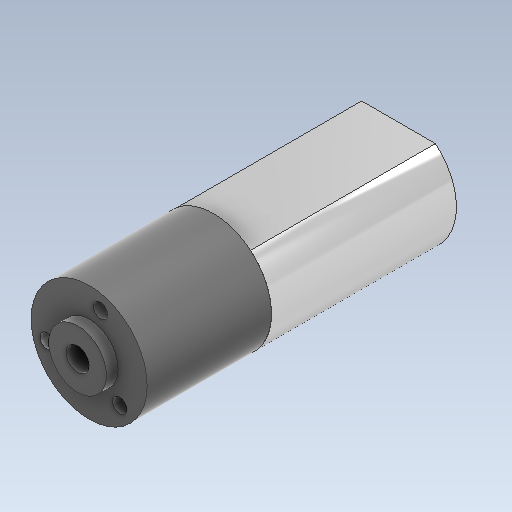
# Autodesk Inventor part: motor_body
Saved by Autodesk Inventor 2020 (Build 240168000, 168)
## iProperties
Created: 2023-12-19
Part Number: motor_body
Material: Типовые
Document SubType Name: Modeling
Designer: denis
Density: 1 g/cm^3
Appearance: По умолчанию
Author: denis
Autodesk Inventor part; units mm, degrees
ref_plane "YZ Plane" through (0, 0, 0) normal (1, 0, 0) x (0, 1, 0)
ref_plane "XZ Plane" through (0, 0, 0) normal (0, 1, 0) x (-1, 0, 0)
ref_plane "XY Plane" through (0, 0, 0) normal (0, 0, 1) x (1, 0, 0)
sketch "Эскиз1" plane through (0, 0, 0) normal (0, 0, 1) x (1, 0, 0)
  circle A0 centre (0, 0) radius 10.025
  dimension "d0" = 20.05
  constraints: 1 centre point, 1 coincident
  measures "d0" diameter of A0
extrude "Выдавливание1" add sketch "Эскиз1" along normal blind 21.5
sketch "Эскиз2" plane through (0, 0, 21.5) normal (0, 0, 1) x (1, 0, 0)
  circle A0 centre (0, 0) radius 5
  dimension "d3" = 10
  constraints: 1 centre point, 1 coincident
  measures "d3" diameter of A0
extrude "Выдавливание2" add sketch "Эскиз2" along normal blind 2
sketch "Эскиз3" plane through (0, 0, 0) normal (0, 0, -1) x (-1, 0, 0)
  circle A0 centre (0, 0) radius 10
  line L0 (6.3804, -7.7) -> (-6.4196, -7.7)
  circle A1 centre (0, 0) radius 10.025 construction
  line L1 (-10.025, 0) -> (10.025, 0) construction
  circle A2 centre (0, 0) radius 10.025 construction
  line L2 (6.3804, 7.7) -> (-6.4196, 7.7)
  point P0 (-6.3804, 7.7)
  point P1 (-6.3804, -7.7)
  dimension "d6" = 20
  dimension "d10" = 15.4
  constraints: 6 end point, 5 point on circle, 2 horizontal, 2 symmetric about line, 1 centre point, 1 coincident
  measures "d6" diameter of A0
  measures "d10" distance between parallel lines of L0 L2
extrude "Выдавливание3" add sketch "Эскиз3" along normal blind 32 contours A0 L0 L2
sketch "Эскиз4" plane through (0, 0, 21.5) normal (0, 0, 1) x (1, 0, 0)
  circle A0 centre (0, 0) radius 7.5 construction
  circle A1 centre (1.9411, 7.2444) radius 1.25
  circle A2 centre (0, 0) radius 10.025 construction
  line L0 (0, 10.025) -> (0, -10.025) construction
  line L1 (1.9411, 7.2444) -> (0, 0) construction
  circle A3 centre (-7.2444, -1.9411) radius 1.25
  circle A4 centre (5.3033, -5.3033) radius 1.25
  dimension "d11" = 15
  dimension "d12" = 2.5
  dimension "d13" = 15
  dimension "d16" = 360
  constraints: 4 end point, 3 centre point, 2 point on circle, 2 vertical, 1 coincident, 10 other
  measures "d12" diameter of A1
  measures "d13" angle of L0 L1
extrude "Выдавливание4" cut sketch "Эскиз4" against normal blind 5
sketch "Эскиз5" plane through (0, 0, -32) normal (0, 0, -1) x (-1, 0, 0)
  circle A0 centre (0, 0) radius 3.1
  dimension "d20" = 6.2
  constraints: 1 centre point, 1 coincident
  measures "d20" diameter of A0
extrude "Выдавливание5" add sketch "Эскиз5" along normal blind 2.1
fillet "Сопряжение1" radius 0.5 1 edges at (3.1, 0, -34.1)
sketch "Эскиз6" plane through (0, 0, -34.1) normal (0, 0, -1) x (-1, 0, 0)
  circle A0 centre (0, 0) radius 1
  dimension "d24" = 2
  constraints: 1 centre point, 1 coincident
  measures "d24" diameter of A0
extrude "Выдавливание6" add sketch "Эскиз6" along normal blind 4.1
sketch "Эскиз7" plane through (0, 0, 23.5) normal (0, 0, 1) x (1, 0, 0)
  circle A0 centre (0, 0) radius 2
  dimension "d27" = 4
  constraints: 1 centre point, 1 coincident
  measures "d27" diameter of A0
extrude "Выдавливание7" cut sketch "Эскиз7" against normal blind 10
